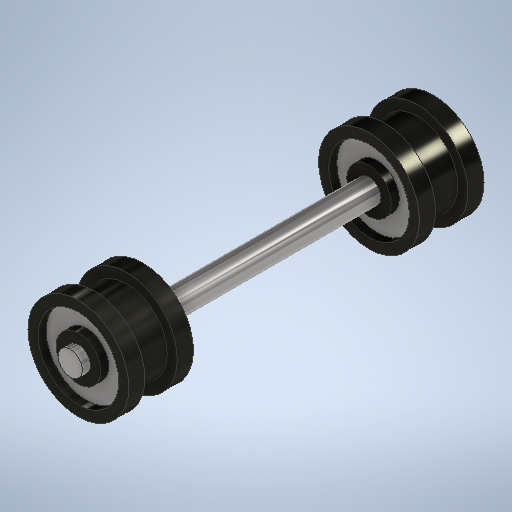
# Autodesk Inventor part: Small Wheels for Polar Express [Copy]
Saved by Autodesk Inventor 2025.1 (Build 291241020, 241B)
## iProperties
Created: 2022-11-29
Part Number: Small Wheels for Polar Express [Copy]
Material: Generic
Document SubType Name: Modeling
Designer: mc_vlongo24
Density: 1 g/cm^3
Appearance: Default
Author: mc_vlongo24
Autodesk Inventor part; units mm, degrees
ref_plane "YZ Plane" through (0, 0, 0) normal (1, 0, 0) x (0, 1, 0)
sketch "Sketch3" plane through (0, 0, 0) normal (0, 0, 1) x (1, 0, 0)
  circle A0 centre (0, 0) radius 6.35
  dimension "d11" = 12.7
  constraints: 1 centre point, 1 coincident
  measures "d11" diameter of A0
extrude "Extrusion3" add sketch "Sketch3" along normal blind 7.62
sketch "Sketch4" plane through (0, 0, 7.62) normal (0, 0, 1) x (1, 0, 0)
  circle A0 centre (0, 0) radius 7.9375
  circle A1 centre (0, 0) radius 6.35
  dimension "d14" = 15.875
  dimension "d15" = 12.7
  constraints: 2 centre point, 2 coincident
  measures "d14" diameter of A0
  measures "d15" diameter of A1
extrude "Extrusion4" add sketch "Sketch4" along normal blind 1.27 and the other way blind 8.89
ref_plane "Work Plane1" through (0, 0, 3.81) normal (0, 0, 1) x (1, 0, 0)
sketch "Sketch5" plane through (0, 0, 3.81) normal (0, 0, 1) x (1, 0, 0)
  circle A0 centre (0, 0) radius 6.35 projected
  circle A1 centre (0, 0) radius 8.89
  circle A2 centre (0, 0) radius 7.9375 projected
  circle A3 centre (0, 0) radius 8.9298
  constraints: 2 centre point, 2 coincident
extrude "Extrusion5" cut sketch "Sketch5" along normal mid plane 5.08 contours A2
sketch "Sketch6" plane through (0, 0, 7.62) normal (0, 0, 1) x (1, 0, 0)
  circle A0 centre (0, 0) radius 1.905
  circle A1 centre (0, 0) radius 3.4925
  dimension "d23" = 3.81
  dimension "d24" = 6.985
  constraints: 2 centre point, 2 coincident
  measures "d23" diameter of A0
  measures "d24" diameter of A1
extrude "Extrusion6" add sketch "Sketch6" along normal blind 1.27 and the other way blind 8.89
sketch "Sketch7" plane through (0, 0, 7.62) normal (0, 0, 1) x (1, 0, 0)
  circle A0 centre (0, 0) radius 3.175
  constraints: 1 centre point, 1 coincident
extrude "Extrusion7" cut sketch "Sketch7" against normal blind 9.2075
sketch "Sketch8" plane through (0, 0, 3.81) normal (0, 0, 1) x (1, 0, 0)
  circle A0 centre (0, 0) radius 1.905
  dimension "d36" = 3.81
  constraints: 1 centre point, 1 coincident
  measures "d36" diameter of A0
extrude "Extrusion8" add sketch "Sketch8" along normal blind 6.35 and the other way blind 22.86
ref_plane "Work Plane2" through (0, 0, -19.05) normal (0, 0, -1) x (-1, 0, 0)
mirror "Mirror1" about plane through (0, 0, -19.05) normal (0, 0, -1) of "Extrusion5", "Extrusion4", "Extrusion3", "Extrusion8", "Extrusion6"
body "Solid2"
